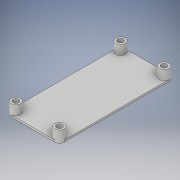
# Autodesk Inventor part: DC converter base
Saved by Autodesk Inventor 2019 (Build 230136000, 136)
## iProperties
Created: 2019-02-10
Part Number: DC converter base
Material: Generic
Document SubType Name: Modeling
Designer: mashimaro
Density: 1 g/cm^3
Appearance: Default
Author: mashimaro
Autodesk Inventor part; units mm, degrees
ref_plane "YZ Plane" through (0, 0, 0) normal (1, 0, 0) x (0, 1, 0)
ref_plane "XZ Plane" through (0, 0, 0) normal (0, 1, 0) x (-1, 0, 0)
ref_plane "XY Plane" through (0, 0, 0) normal (0, 0, 1) x (1, 0, 0)
sketch "Sketch1" plane through (0, 0, 0) normal (0, 1, 0) x (-1, 0, 0)
  arc A0 (13.9, 27.4) -> (11.4, 29.9) centre (11.4, 27.4) ccw
  arc A1 (-11.4, 29.9) -> (-13.9, 27.4) centre (-11.4, 27.4) ccw
  arc A2 (11.4, -29.9) -> (13.9, -27.4) centre (11.4, -27.4) ccw
  arc A3 (-13.9, -27.4) -> (-11.4, -29.9) centre (-11.4, -27.4) ccw
  line L0 (11.4, 29.9) -> (-11.4, 29.9)
  line L1 (-13.9, 27.4) -> (-13.9, -27.4)
  line L2 (-11.4, -29.9) -> (11.4, -29.9)
  line L3 (13.9, -27.4) -> (13.9, 27.4)
  point P0 (0, 0)
  constraints: 8 end point, 8 point on circle, 5 tangent, 4 centre point, 1 perpendicular
extrude "Extrusion1" add sketch "Sketch1" along normal blind 1
sketch "Sketch2" plane through (0, 1, 0) normal (0, 1, 0) x (1, 0, 0)
  arc A0 (-13.9, -27.4) -> (-11.4, -29.9) centre (-11.4, -27.4) ccw projected
  circle A1 centre (-11.4, -27.4) radius 2.5
  circle A2 centre (-11.4, -27.4) radius 1.5
  arc A3 (11.4, -29.9) -> (13.9, -27.4) centre (11.4, -27.4) ccw projected
  circle A4 centre (11.4, -27.4) radius 2.5
  circle A5 centre (11.4, -27.4) radius 1.5
  arc A6 (13.9, 27.4) -> (11.4, 29.9) centre (11.4, 27.4) ccw projected
  circle A7 centre (11.4, 27.4) radius 2.5
  circle A8 centre (11.4, 27.4) radius 1.5
  arc A9 (-11.4, 29.9) -> (-13.9, 27.4) centre (-11.4, 27.4) ccw projected
  circle A10 centre (-11.4, 27.4) radius 2.5
  circle A11 centre (-11.4, 27.4) radius 1.5
  point P0 (0, 0)
  dimension "d17" = 3
  dimension "d18" = 3
  dimension "d19" = 3
  dimension "d20" = 3
  constraints: 8 coincident, 5 centre point, 2 horizontal alignment, 1 vertical alignment, 6 other
  measures "d17" diameter of A2
  measures "d18" diameter of A5
  measures "d19" diameter of A8
  measures "d20" diameter of A11
extrude "Extrusion2" add sketch "Sketch2" along normal blind 5
body "Solid1"
